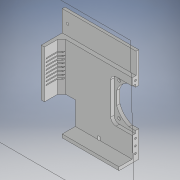
# Autodesk Inventor part: 000.001.009 - Накладка центральная
Saved by Autodesk Inventor 2022 (Build 260153000, 153)
## iProperties
Created: 2022-12-25
Part Number: 000.001.009 - Накладка центральная
Material: Типовые
Document SubType Name: Modeling
Designer: Ivan Petrov
Density: 1 g/cm^3
Appearance: По умолчанию
Mass: 265.631 g
Surface Area: 795.027 cm^2
Volume: 265.631 cm^3
Author: Ivan Petrov
Autodesk Inventor part; units mm, degrees
ref_plane "YZ Plane" through (0, 0, 0) normal (1, 0, 0) x (0, 1, 0)
ref_plane "XZ Plane" through (0, 0, 0) normal (0, 1, 0) x (-1, 0, 0)
ref_plane "XY Plane" through (0, 0, 0) normal (0, 0, 1) x (1, 0, 0)
sketch "Эскиз1" plane through (0, 0, 0) normal (0, 0, 1) x (1, 0, 0)
  line L0 (5.3151, -72.5414) -> (177.8151, -72.5414) projected
  line L1 (177.8151, -152.5414) -> (177.8151, -32.5414) projected
  line L2 (5.3151, -152.5414) -> (5.3151, -32.5414) projected
  line L3 (5.3151, -32.5414) -> (-4.6849, -32.5414) projected
  line L4 (-49.9349, -32.5414) -> (-4.6849, -32.5414) projected
  line L5 (-20.4349, 12.1553) -> (-20.4349, 32.2619) projected
  line L6 (-20.4349, 12.1553) -> (-20.4349, 9.9586) projected
  line L7 (-20.4349, 37.5652) -> (-20.4349, 32.2619) projected
  line L8 (-20.4349, 37.5652) -> (-20.4349, 39.4586) projected
  line L9 (235.5651, 39.4586) -> (-52.4349, 39.4586) projected
  line L10 (177.8151, -32.5414) -> (187.8151, -32.5414) projected
  line L11 (233.0651, -32.5414) -> (187.8151, -32.5414) projected
  line L12 (203.5651, 9.9586) -> (203.5651, 12.1553) projected
  line L13 (203.5651, 12.1553) -> (203.5651, 32.2619) projected
  line L14 (203.5651, 32.2619) -> (203.5651, 37.5652) projected
  line L15 (203.5651, 37.5652) -> (203.5651, 39.4586) projected
  line L16 (203.5651, 12.1553) -> (203.5651, 32.2619) projected
  line L17 (203.5651, 12.1553) -> (203.5651, 32.2619) projected
  line L18 (-20.4349, 9.9586) -> (-20.4349, -32.5414)
  line L19 (203.5651, 9.9586) -> (203.5651, -32.5414)
  point P0 (0, 0)
  constraints: 4 end point, 2 vertical, 4 other
extrude "Выдавливание1" add sketch "Эскиз1" along normal blind 10
sketch "Эскиз7" plane through (0, 0, 10) normal (0, 0, 1) x (1, 0, 0)
  line L0 (-20.4349, 39.4586) -> (-20.4349, -32.5414) projected
  line L1 (-20.4349, -32.5414) -> (5.3151, -32.5414) projected
  line L2 (-20.4349, 39.4586) -> (-15.4349, 39.4586)
  line L3 (-15.4349, 39.4586) -> (-15.4349, -32.5414)
  line L4 (-15.4349, -32.5414) -> (-20.4349, -32.5414)
  line L5 (-20.4349, -32.5414) -> (-20.4349, 39.4586)
  line L6 (203.5651, -32.5414) -> (203.5651, 39.4586) projected
  line L7 (177.8151, -32.5414) -> (203.5651, -32.5414) projected
  line L8 (203.5651, 39.4586) -> (198.5651, 39.4586)
  line L9 (198.5651, 39.4586) -> (198.5651, -32.5414)
  line L10 (198.5651, -32.5414) -> (203.5651, -32.5414)
  line L11 (203.5651, -32.5414) -> (203.5651, 39.4586)
  point P0 (0, 0)
  point P1 (-19.4349, 9.9586)
  point P2 (5.3151, -32.5414)
  point P3 (202.5651, 9.9586)
  dimension "d13" = 5
  dimension "d14" = 5
  constraints: 16 end point, 4 parallel, 2 horizontal, 2 perpendicular, 6 other
  measures "d13" distance of L3.end L4.end
  measures "d14" distance of L10.end L9.end
extrude "Выдавливание6" add sketch "Эскиз7" along normal blind 26
sketch "Эскиз10" plane through (0, 0, 10) normal (0, 0, 1) x (1, 0, 0)
  line L0 (5.3151, -72.5414) -> (177.8151, -72.5414) projected
  line L1 (177.8151, -72.5414) -> (177.8151, -32.5414) projected
  line L2 (5.3151, -72.5414) -> (177.8151, -72.5414)
  line L3 (177.8151, -72.5414) -> (177.8151, -67.5414)
  line L4 (177.8151, -67.5414) -> (5.3151, -67.5414)
  line L5 (5.3151, -67.5414) -> (5.3151, -72.5414)
  point P0 (0, 0)
  dimension "d23" = 5
  constraints: 8 end point, 2 parallel, 1 horizontal, 1 perpendicular, 1 point on line
  measures "d23" distance of L3.end L2.end
extrude "Выдавливание9" add sketch "Эскиз10" along normal blind 20
sketch "Эскиз11" plane through (-20.4349, 39.4586, 0) normal (0, 1, 0) x (1, 0, 0)
  line L0 (224, 0) -> (224, -36) projected
  line L1 (0, 0) -> (224, 0)
  line L2 (224, 0) -> (224, -4)
  line L3 (224, -4) -> (0, -4)
  line L4 (0, -4) -> (0, 0)
  point P0 (20.4349, 0)
  dimension "d26" = 4
  constraints: 8 end point, 2 parallel, 1 horizontal, 1 perpendicular, 1 point on line
  measures "d26" distance between parallel lines of L3 L1
extrude "Выдавливание10" add sketch "Эскиз11" along normal blind 32
sketch "Эскиз12" plane through (5.3151, -72.5414, 0) normal (0, -1, 0) x (1, 0, 0)
  circle A0 centre (36.25, 8) radius 2.75 projected
  circle A1 centre (136.25, 8) radius 2.75 projected
  point P0 (-5.3151, 0)
extrude "Выдавливание11" cut sketch "Эскиз12" against normal blind 10
sketch "Эскиз13" plane through (0, 0, 0) normal (0, 0, -1) x (-1, 0, 0)
  circle A0 centre (12.4349, 55.4586) radius 1.85 projected
  circle A1 centre (-195.5651, 55.4586) radius 1.85 projected
  point P0 (0, 0)
extrude "Выдавливание12" cut sketch "Эскиз13" against normal blind 10
sketch "Эскиз15" plane through (0, 0, 0) normal (0, 0, -1) x (-1, 0, 0)
  circle A0 centre (-66.5651, -28.8688) radius 2.25 projected
  circle A1 centre (-66.5651, 21.1312) radius 2.25 projected
  circle A2 centre (-116.5651, 21.1312) radius 2.25 projected
  circle A3 centre (-116.5651, -28.8688) radius 2.25 projected
  circle A4 centre (-91.5651, -3.8688) radius 14 projected
  arc A5 (-121.5651, -28.3688) -> (-116.0651, -33.8688) centre (-116.0651, -28.3688) ccw
  line L0 (-67.0651, -33.8688) -> (-116.0651, -33.8688)
  arc A6 (-67.0651, -33.8688) -> (-61.5651, -28.3688) centre (-67.0651, -28.3688) ccw
  line L1 (-61.5651, 20.6312) -> (-61.5651, -28.3688)
  arc A7 (-61.5651, 20.6312) -> (-67.0651, 26.1312) centre (-67.0651, 20.6312) ccw
  line L2 (-116.0651, 26.1312) -> (-67.0651, 26.1312)
  arc A8 (-116.0651, 26.1312) -> (-121.5651, 20.6312) centre (-116.0651, 20.6312) ccw
  line L3 (-121.5651, -28.3688) -> (-121.5651, 20.6312)
  arc A9 (-73.2286, 20.1316) -> (-81.5651, 24.6312) centre (-91.5651, -3.8688) ccw
  arc A10 (-101.5651, 24.6312) -> (-113.4494, 16.9478) centre (-91.5651, -3.8688) ccw
  line L4 (-81.5651, 24.6312) -> (-101.5651, 24.6312)
  arc A11 (-101.5651, 24.6312) -> (-120.0651, 6.1312) centre (-91.5651, -3.8688) ccw
  arc A12 (-120.0651, -13.8688) -> (-101.5651, -32.3688) centre (-91.5651, -3.8688) ccw
  line L5 (-120.0651, 6.1312) -> (-120.0651, -13.8688)
  arc A13 (-116.0609, -21.5382) -> (-101.5651, -32.3688) centre (-91.5651, -3.8688) ccw
  arc A14 (-81.5651, -32.3688) -> (-63.0651, -13.8688) centre (-91.5651, -3.8688) ccw
  line L6 (-81.5651, -32.3688) -> (-101.5651, -32.3688)
  circle A15 centre (-116.5651, -28.8688) radius 2.25
  circle A16 centre (-66.5651, -28.8688) radius 2.25
  circle A17 centre (-66.5651, 21.1312) radius 2.25
  arc A18 (-63.0651, 6.1312) -> (-81.5651, 24.6312) centre (-91.5651, -3.8688) ccw
  line L7 (-63.0651, 6.1312) -> (-63.0651, -13.8688)
  arc A19 (-67.5275, -22.1566) -> (-63.0651, -13.8688) centre (-91.5651, -3.8688) ccw
  circle A20 centre (-116.5651, 21.1312) radius 2.25
  point P0 (0, 0)
  point P1 (-113.4494, 16.9478)
  point P2 (-73.2286, 20.1316)
  constraints: 24 point on circle, 16 centre point, 16 end point
extrude "Выдавливание13" cut sketch "Эскиз15" against normal blind 10 contours A0 | A1 | A2 | A3 | A4 | A18 L7 A14 L6 A12 L5 A11 A10 L4 A9
chamfer "Фаска1" distance 3 angle 45 4 edges at (68.8151, 21.1312, 0) (68.8151, -28.8688, 0) (118.8151, -28.8688, 0) (118.8151, 21.1312, 0)
sketch "Эскиз16" plane through (0, 0, 10) normal (0, 0, 1) x (1, 0, 0)
  circle A0 centre (66.5651, 21.1312) radius 2.25
  circle A1 centre (116.5651, 21.1312) radius 2.25
  circle A2 centre (116.5651, -28.8688) radius 2.25
  circle A3 centre (66.5651, -28.8688) radius 2.25
  line L0 (61.5651, -28.3688) -> (61.5651, 20.6312)
  arc A4 (67.0651, 26.1312) -> (61.5651, 20.6312) centre (67.0651, 20.6312) ccw
  line L1 (67.0651, 26.1312) -> (116.0651, 26.1312)
  arc A5 (121.5651, 20.6312) -> (116.0651, 26.1312) centre (116.0651, 20.6312) ccw
  line L2 (121.5651, 20.6312) -> (121.5651, -28.3688)
  arc A6 (116.0651, -33.8688) -> (121.5651, -28.3688) centre (116.0651, -28.3688) ccw
  line L3 (116.0651, -33.8688) -> (67.0651, -33.8688)
  arc A7 (61.5651, -28.3688) -> (67.0651, -33.8688) centre (67.0651, -28.3688) ccw
  arc A8 (120.0651, 6.1312) -> (101.5651, 24.6312) centre (91.5651, -3.8688) ccw projected
  arc A9 (81.5651, 24.6312) -> (63.0651, 6.1312) centre (91.5651, -3.8688) ccw projected
  point P0 (0, 0)
  constraints: 8 centre point, 8 end point, 8 point on circle
extrude "Выдавливание14" cut sketch "Эскиз16" against normal blind 5 contours A0 | A1 | A2 | A3 | L0 A4 L1 A5 L2 A6 L3 A7
sketch "Эскиз17" plane through (177.8151, -32.5414, 0) normal (0, -1, 0) x (1, 0, 0)
  line L0 (25.75, 0) -> (25.75, 36) projected
  line L1 (0, 0) -> (25.75, 0) projected
  line L2 (55.25, 36) -> (10, 0) projected
  point P0 (-177.8151, 0)
  point P1 (25.75, 12.5304)
extrude "Выдавливание15" cut sketch "Эскиз17" against normal blind 40
chamfer "Фаска2" distance 6.5 angle 45 2 edges at (198.5651, 3.4586, 10) (-15.4349, 3.4586, 10)
ref_plane "РабПлоскость1" through (91.5651, 71.4586, 0) normal (1, 0, 0) x (0, 0, -1)
draft "НаклГрань1" angle 72.6 pull direction (0, 0, -1) faces at (198.3151, 7.4586, 4.1768) fixed edges at (195.6901, 7.4586, 0)
sketch "Эскиз18" plane through (203.5651, -32.5414, 36) normal (1, 0, 0) x (0, 0, -1)
  line L0 (25.2856, 21.5321) -> (3.2856, 21.5321)
  line L1 (3.2856, 21.5321) -> (2, 20)
  line L2 (2, 20) -> (24, 20)
  line L3 (24, 20) -> (25.2856, 21.5321)
  line L4 (23.4696, 0) -> (0, 0) projected
  line L5 (0, 0) -> (0, 72) projected
  point P0 (36, 32.5414)
  dimension "d46" = 50
  dimension "d47" = 2
  dimension "d48" = 22
  dimension "d49" = 20
  dimension "d50" = 2
  constraints: 8 end point, 2 parallel, 1 horizontal
  measures "d46" angle of L2 L1
  measures "d47" distance of L2.end L0.start
  measures "d48" distance of L0.start L0.end
  measures "d49" distance between parallel lines of L4 L2
  measures "d50" distance from line of L5 L1.end
extrude "Выдавливание16" cut sketch "Эскиз18" against normal blind 14
pattern_linear "Прямоуг.массив1" count 8 spacing 5 along (0, 1, 0) of "Выдавливание16"
mirror "Зеркальное отражение2" about plane through (91.5651, 71.4586, 0) normal (1, 0, 0) of "Выдавливание15"
draft "НаклГрань2" angle 72.6 pull direction (0, 0, -1) faces at (-15.1849, 7.4586, 4.1768) fixed edges at (-12.5599, 7.4586, 0)
mirror "Зеркальное отражение3" about plane through (91.5651, 71.4586, 0) normal (1, 0, 0) of "Выдавливание16", "Прямоуг.массив1"
offset faces "Размер1" outward -2.5 faces at (118.0745, -33.4886, 6.6667) (83.3985, -33.8688, 8.3333) (65.0558, -33.4886, 6.6667) (61.5651, 4.2978, 8.3333) (121.5651, -12.0355, 8.3333) (119.8061, 24.663, 6.6667) (99.7318, 26.1312, 8.3333) (65.0558, 25.751, 6.6667)
sketch "Эскиз19" plane through (0, 0, 10) normal (0, 0, 1) x (1, 0, 0)
  circle A0 centre (116.5651, 21.1312) radius 2.25 projected
  circle A1 centre (116.5651, -28.8688) radius 2.25 projected
  arc A2 (63.0651, -13.8688) -> (81.5651, -32.3688) centre (91.5651, -3.8688) ccw projected
  line L0 (63.0651, 6.1312) -> (63.0651, -13.8688) projected
  arc A3 (81.5651, 24.6312) -> (63.0651, 6.1312) centre (91.5651, -3.8688) ccw projected
  line L1 (101.5651, 24.6312) -> (81.5651, 24.6312) projected
  arc A4 (120.0651, 6.1312) -> (101.5651, 24.6312) centre (91.5651, -3.8688) ccw projected
  line L2 (120.0651, -13.8688) -> (120.0651, 6.1312) projected
  arc A5 (101.5651, -32.3688) -> (120.0651, -13.8688) centre (91.5651, -3.8688) ccw projected
  line L3 (81.5651, -32.3688) -> (101.5651, -32.3688) projected
  circle A6 centre (66.5651, -28.8688) radius 2.25 projected
  circle A7 centre (66.5651, 21.1312) radius 2.25 projected
  line L4 (124.0651, 20.6312) -> (124.0651, -28.3688) projected
  arc A8 (124.0651, 20.6312) -> (116.0651, 28.6312) centre (116.0651, 20.6312) ccw projected
  line L5 (67.0651, 28.6312) -> (116.0651, 28.6312) projected
  arc A9 (67.0651, 28.6312) -> (59.0651, 20.6312) centre (67.0651, 20.6312) ccw projected
  line L6 (59.0651, -28.3688) -> (59.0651, 20.6312) projected
  arc A10 (59.0651, -28.3688) -> (67.0651, -36.3688) centre (67.0651, -28.3688) ccw projected
  line L7 (116.0651, -36.3688) -> (67.0651, -36.3688) projected
  arc A11 (116.0651, -36.3688) -> (124.0651, -28.3688) centre (116.0651, -28.3688) ccw projected
  line L8 (-8.9349, -32.5414) -> (-8.9349, 39.4586) projected
  line L9 (-8.9349, -32.5414) -> (5.3151, -32.5414) projected
  line L10 (5.3151, -32.5414) -> (5.3151, -67.5414) projected
  line L11 (5.3151, -67.5414) -> (39.6777, -67.5414) projected
  line L12 (39.6777, -67.5414) -> (39.6777, -62.5414) projected
  line L13 (39.6777, -62.5414) -> (43.4526, -62.5414) projected
  line L14 (43.4526, -62.5414) -> (43.4526, -67.5414) projected
  line L15 (43.4526, -67.5414) -> (139.6777, -67.5414) projected
  line L16 (139.6777, -67.5414) -> (139.6777, -62.5414) projected
  line L17 (139.6777, -62.5414) -> (143.4526, -62.5414) projected
  line L18 (143.4526, -62.5414) -> (143.4526, -67.5414) projected
  line L19 (143.4526, -67.5414) -> (177.8151, -67.5414) projected
  line L20 (177.8151, -67.5414) -> (177.8151, -32.5414) projected
  line L21 (177.8151, -32.5414) -> (192.0651, -32.5414) projected
  line L22 (192.0651, 39.4586) -> (192.0651, -32.5414) projected
  line L23 (192.0651, 39.4586) -> (-8.9349, 39.4586) projected
  arc A12 (124.0651, 20.6312) -> (116.0651, 28.6312) centre (116.0651, 20.6312) ccw projected
  line L24 (124.0651, 20.6312) -> (124.0651, -28.3688) projected
  arc A13 (116.0651, -36.3688) -> (124.0651, -28.3688) centre (116.0651, -28.3688) ccw projected
  line L25 (116.0651, -36.3688) -> (67.0651, -36.3688) projected
  arc A14 (59.0651, -28.3688) -> (67.0651, -36.3688) centre (67.0651, -28.3688) ccw projected
  line L26 (59.0651, -28.3688) -> (59.0651, 20.6312) projected
  arc A15 (67.0651, 28.6312) -> (59.0651, 20.6312) centre (67.0651, 20.6312) ccw projected
  line L27 (67.0651, 28.6312) -> (116.0651, 28.6312) projected
  point P0 (0, 0)
ref_plane "РабПлоскость2" through (91.5651, 24.6312, 5) normal (1, 0, 0) x (0, 0, -1)
sketch "Эскиз20" plane through (91.5651, 24.6312, 5) normal (1, 0, 0) x (0, 0, -1)
  line L0 (-87.0101, 83.0756) -> (41.4391, 83.0756)
  line L1 (41.4391, 83.0756) -> (41.4391, -122.5086)
  line L2 (41.4391, -122.5086) -> (-87.0101, -122.5086)
  line L3 (-87.0101, -122.5086) -> (-87.0101, 83.0756)
  point P0 (5, -24.6312)
  constraints: 8 end point, 2 parallel, 1 horizontal, 1 perpendicular
extrude "Выдавливание17" cut sketch "Эскиз20" along normal through all
sketch "Эскиз21" plane through (91.5651, 24.6312, 5) normal (1, 0, 0) x (0, 0, -1)
  circle A0 centre (0, -87.1726) radius 1.5
  line L0 (5, -97.1726) -> (-25, -97.1726) projected
  point P0 (5, -24.6312)
  point P1 (0, -57)
  dimension "d60" = 3
  dimension "d61" = 10
  constraints: 1 centre point, 1 vertical alignment
  measures "d60" diameter of A0
  measures "d61" distance from line of L0 A0.centre
extrude "Выдавливание18" cut sketch "Эскиз21" against normal blind 10
pattern_linear "Прямоуг.массив2" count 3 spacing 10 along (0, 1, 0) of "Выдавливание18"
sketch "Эскиз22" plane through (91.5651, 24.6312, 5) normal (1, 0, 0) x (0, 0, -1)
  circle A0 centre (0, 8.8274) radius 1.5
  line L0 (-5, 14.8274) -> (1, 14.8274) projected
  point P0 (5, -24.6312)
  point P1 (0, 4)
  dimension "d67" = 3
  dimension "d68" = 6
  constraints: 1 centre point, 1 vertical alignment
  measures "d67" diameter of A0
  measures "d68" distance from line of L0 A0.centre
extrude "Выдавливание19" cut sketch "Эскиз22" against normal blind 10
